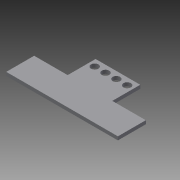
# Autodesk Inventor part: Mount Motor
Saved by Autodesk Inventor 2013 (Build 170138000, 138)
## iProperties
Created: 2013-01-21
Part Number: Mount Motor
Material: Generic
Document SubType Name: Modeling
Designer: actoennies
Density: 1 g/cm^3
Author: actoennies
Autodesk Inventor part; units mm, degrees
ref_plane "YZ Plane" through (0, 0, 0) normal (1, 0, 0) x (0, 1, 0)
ref_plane "XZ Plane" through (0, 0, 0) normal (0, 1, 0) x (-1, 0, 0)
ref_plane "XY Plane" through (0, 0, 0) normal (0, 0, 1) x (1, 0, 0)
sketch "Sketch1" plane through (0, 0, 0) normal (0, 1, 0) x (-1, 0, 0)
  circle A0 centre (-131.2765, -95.25) radius 3.3782
  circle A1 centre (-141.1255, -95.25) radius 3.3782
  circle A2 centre (-150.9745, -95.25) radius 3.3782
  circle A3 centre (-160.8235, -95.25) radius 3.3782
  line L0 (-146.05, -156.4252) -> (-146.05, 317.5689) construction
  line L1 (-125.73, -156.4252) -> (-125.73, 317.5689) construction
  line L2 (-166.37, -156.4252) -> (-166.37, 317.5689) construction
  line L3 (-166.37, -101.6) -> (-166.37, -76.2)
  line L4 (-166.37, -76.2) -> (-196.85, -76.2)
  line L5 (-196.85, -76.2) -> (-196.85, -50.8)
  line L6 (-196.85, -50.8) -> (-95.25, -50.8)
  line L7 (-95.25, -50.8) -> (-95.25, -76.2)
  line L8 (-95.25, -76.2) -> (-125.73, -76.2)
  line L9 (-125.73, -76.2) -> (-125.73, -101.6)
  line L10 (-166.37, -101.6) -> (-125.73, -101.6)
  dimension "d4" = 20.32
  dimension "d5" = 20.32
  dimension "d6" = 25.4
  dimension "d7" = 30.48
  dimension "d8" = 25.4
  dimension "d9" = 101.6
  dimension "d10" = 30.48
  constraints: 22 end point, 4 centre point, 4 perpendicular, 4 point on line, 3 parallel, 8 other
  measures "d4" distance between parallel lines of L1 L0
  measures "d5" distance between parallel lines of L2 L0
  measures "d6" distance of L3.start L3.end
  measures "d7" distance of L3.end L4.end
  measures "d8" distance of L4.end L5.end
  measures "d9" distance of L5.end L6.end
  measures "d10" distance of L7.end L8.end
extrude "Extrusion1" add sketch "Sketch1" along normal blind 3.175
body "Solid1"
